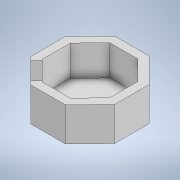
# Autodesk Inventor part: TokenHolderSingle
Saved by Autodesk Inventor 2020 (Build 240168000, 168)
## iProperties
Created: 2020-06-16
Part Number: TokenHolderSingle
Material: Generic
Document SubType Name: Modeling
Designer: user
Density: 1 g/cm^3
Appearance: Default
Author: user
## iProperties of the stored document _3DPrint.ipt
Created: 2020-06-16
Part Number: _3DPrint
Material: Generic
Document SubType Name: Modeling
Designer: user
Density: 1 g/cm^3
Appearance: Default
Author: user
Autodesk Inventor part; units mm, degrees
ref_plane "YZ Plane" through (0, 0, 0) normal (1, 0, 0) x (0, 1, 0)
ref_plane "XZ Plane" through (0, 0, 0) normal (0, 1, 0) x (-1, 0, 0)
ref_plane "XY Plane" through (0, 0, 0) normal (0, 0, 1) x (1, 0, 0)
sketch "Sketch1" plane through (0, 0, 0) normal (0, 1, 0) x (-1, 0, 0)
  line L0 (7.5264, 21.8341) -> (7.5264, 13.5841)
  line L1 (7.5264, 13.5841) -> (1.7974, 7.6477)
  line L2 (1.7974, 7.6477) -> (-6.4526, 7.6477)
  line L3 (7.5264, 21.8341) -> (1.6928, 27.6678)
  line L4 (1.6928, 27.6678) -> (-6.5572, 27.6678)
  line L5 (-6.5572, 27.6678) -> (-12.2862, 21.7314)
  line L6 (-12.2862, 21.7314) -> (-12.2862, 13.4814)
  line L7 (-12.2862, 13.4814) -> (-6.4526, 7.6477)
  line L8 (9.9412, 22.8339) -> (9.9412, 12.5839)
  line L9 (9.9412, 12.5839) -> (2.7976, 5.2333)
  line L10 (2.7976, 5.2333) -> (-7.4524, 5.2333)
  line L11 (9.9412, 22.8339) -> (2.6934, 30.0818)
  line L12 (2.6934, 30.0818) -> (-7.5566, 30.0818)
  line L13 (-7.5566, 30.0818) -> (-14.7002, 22.7311)
  line L14 (-14.7002, 22.7311) -> (-14.7002, 12.4811)
  line L15 (-14.7002, 12.4811) -> (-7.4524, 5.2333)
  point P0 (0, 0)
  point P1 (1, 1)
  dimension "d0" = 8.25
  dimension "d3" = 8.25
  dimension "d5" = 8.25
  dimension "d7" = 8.25
  dimension "d8" = 8.25
  dimension "d9" = 8.25
  dimension "d12" = 8.25
  dimension "d17" = 8.25
  dimension "d18" = 135
  dimension "d19" = 10.25
  dimension "d20" = 10.25
  dimension "d21" = 10.25
  dimension "d22" = 10.25
  dimension "d23" = 10.25
  dimension "d24" = 10.25
  dimension "d25" = 10.25
  dimension "d26" = 10.25
  dimension "d27" = 135
  dimension "d29" = 2.414
  dimension "d31" = 2.414
  dimension "d32" = 2.4144
  dimension "d33" = 2.4148
  constraints: 32 end point, 4 horizontal, 4 vertical
  measures "d0" distance of L0.end L0.start
  measures "d3" distance of L0.end L1.end
  measures "d5" distance of L1.end L2.end
  measures "d7" distance of L0.start L3.end
  measures "d8" distance of L3.end L4.end
  measures "d9" distance of L4.end L5.end
  measures "d12" distance of L5.end L6.end
  measures "d17" distance of L6.end L2.end
  measures "d18" angle of L0 L3
  measures "d19" distance of L8.end L8.start
  measures "d20" distance of L8.end L9.end
  measures "d21" distance of L9.end L10.end
  measures "d22" distance of L8.start L11.end
  measures "d23" distance of L11.end L12.end
  measures "d24" distance of L12.end L13.end
  measures "d25" distance of L13.end L14.end
  measures "d26" distance of L14.end L10.end
  measures "d27" angle of L8 L11
  measures "d29" distance between parallel lines of L14 L6
  measures "d31" distance between parallel lines of L12 L4
  measures "d32" distance between parallel lines of L10 L2
  measures "d33" distance between parallel lines of L0 L8
extrude "OutsideHeight" add sketch "Sketch1" along normal blind 10
extrude "BaseHeight" add sketch "Sketch1" along normal blind 1 contours L0 L1 L2 L7 L6 L5 L4 L3
sketch "Sketch2" plane through (-2.6934, 0, 30.0818) normal (-0.7071068, 0, 0.7071068) x (0.7071068, 0, 0.7071068)
  line L0 (-10.25, 10) -> (0, 10) projected
  line L1 (-0.1464, 0) -> (-10.3964, 0) projected
  line L2 (-8.75, 10) -> (-1.5, 10)
  line L3 (-10.25, 0) -> (-10.25, 10) projected
  line L4 (0, 0) -> (0, 10) projected
  line L5 (-8.75, 1) -> (-1.5, 1)
  line L6 (-8.75, 10) -> (-8.75, 1)
  line L7 (-1.5, 10) -> (-1.5, 1)
  point P0 (-19.3665, 0)
  dimension "d41" = 1.5
  dimension "d42" = 1.5
  dimension "d43" = 1
  constraints: 8 end point, 2 point on line
  measures "d41" distance between parallel lines of L6 L3
  measures "d42" distance between parallel lines of L4 L7
  measures "d43" distance between parallel lines of L1 L5
extrude "SideCut" cut sketch "Sketch2" against normal blind 2.5
equation "\"d3\" = d0"
equation "\"d5\" = d0"
equation "\"d7\" = d0"
equation "\"d8\" = d0"
equation "\"d9\" = d0"
equation "\"d12\" = d0"
equation "\"d17\" = d0"
equation "\"d20\" = d19"
equation "\"d21\" = d19"
equation "\"d22\" = d19"
equation "\"d23\" = d19"
equation "\"d24\" = d19"
equation "\"d25\" = d19"
equation "\"d26\" = d19"
equation "\"d42\" = d41"
body "Solid1"
